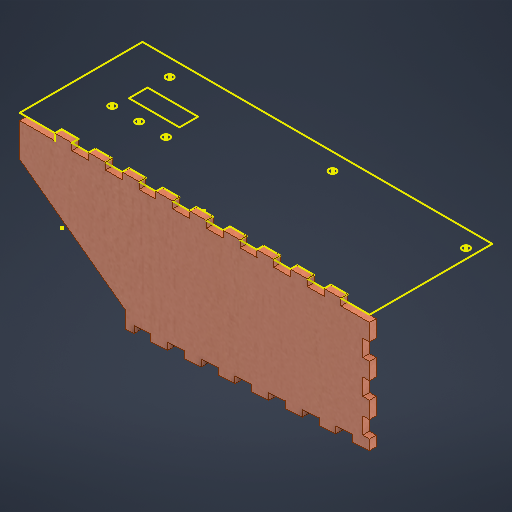
# Autodesk Inventor part: стульчак 2
Saved by Autodesk Inventor 2025 (Build 290162000, 162)
## iProperties
Created: 2025-01-28
Part Number: стульчак 2
Material: Древесина (орех)
Document SubType Name: Modeling
Designer: GameHD
Density: 0.55 g/cm^3
Appearance: Орех — натуральный — полированный
Author: GameHD
Autodesk Inventor part; units mm, degrees
ref_plane "YZ Plane" through (0, 0, 0) normal (1, 0, 0) x (0, 1, 0)
ref_plane "XZ Plane" through (0, 0, 0) normal (0, 1, 0) x (-1, 0, 0)
ref_plane "XY Plane" through (0, 0, 0) normal (0, 0, 1) x (1, 0, 0)
sketch "Эскиз1" plane through (0, 0, 0) normal (0, 0, 1) x (1, 0, 0)
  line L0 (105.5, -51) -> (-105.5, -51)
  line L1 (-105.5, -51) -> (-105.5, 51)
  line L2 (-105.5, 51) -> (105.5, 51)
  line L3 (105.5, 51) -> (105.5, -51)
  line L4 (105.5, -51) -> (-105.5, 51) construction
  line L5 (-105.5, -51) -> (105.5, 51) construction
  line L6 (105.5, 47) -> (-105.5, 47)
  line L7 (105.5, 47) -> (105.5, 51)
  line L8 (105.5, 51) -> (95.5, 51)
  line L9 (95.5, 51) -> (95.5, 47)
  line L10 (95.5, 47) -> (105.5, 47)
  line L11 (85.5, 51) -> (85.5, 47)
  line L12 (95.5, 51) -> (85.5, 51)
  line L13 (95.5, 47) -> (95.5, 51)
  line L14 (85.5, 47) -> (95.5, 47)
  line L15 (75.5, 51) -> (75.5, 47)
  line L16 (85.5, 51) -> (75.5, 51)
  line L17 (85.5, 47) -> (85.5, 51)
  line L18 (75.5, 47) -> (85.5, 47)
  line L19 (65.5, 51) -> (65.5, 47)
  line L20 (75.5, 51) -> (65.5, 51)
  line L21 (75.5, 47) -> (75.5, 51)
  line L22 (65.5, 47) -> (75.5, 47)
  line L23 (55.5, 51) -> (55.5, 47)
  line L24 (65.5, 51) -> (55.5, 51)
  line L25 (65.5, 47) -> (65.5, 51)
  line L26 (55.5, 47) -> (65.5, 47)
  line L27 (45.5, 51) -> (45.5, 47)
  line L28 (55.5, 51) -> (45.5, 51)
  line L29 (55.5, 47) -> (55.5, 51)
  line L30 (45.5, 47) -> (55.5, 47)
  line L31 (35.5, 51) -> (35.5, 47)
  line L32 (45.5, 51) -> (35.5, 51)
  line L33 (45.5, 47) -> (45.5, 51)
  line L34 (35.5, 47) -> (45.5, 47)
  line L35 (25.5, 51) -> (25.5, 47)
  line L36 (35.5, 51) -> (25.5, 51)
  line L37 (35.5, 47) -> (35.5, 51)
  line L38 (25.5, 47) -> (35.5, 47)
  line L39 (15.5, 51) -> (15.5, 47)
  line L40 (25.5, 51) -> (15.5, 51)
  line L41 (25.5, 47) -> (25.5, 51)
  line L42 (15.5, 47) -> (25.5, 47)
  line L43 (5.5, 51) -> (5.5, 47)
  line L44 (15.5, 51) -> (5.5, 51)
  line L45 (15.5, 47) -> (15.5, 51)
  line L46 (5.5, 47) -> (15.5, 47)
  line L47 (-4.5, 51) -> (-4.5, 47)
  line L48 (5.5, 51) -> (-4.5, 51)
  line L49 (5.5, 47) -> (5.5, 51)
  line L50 (-4.5, 47) -> (5.5, 47)
  line L51 (-14.5, 51) -> (-14.5, 47)
  line L52 (-4.5, 51) -> (-14.5, 51)
  line L53 (-4.5, 47) -> (-4.5, 51)
  line L54 (-14.5, 47) -> (-4.5, 47)
  line L55 (-24.5, 51) -> (-24.5, 47)
  line L56 (-14.5, 51) -> (-24.5, 51)
  line L57 (-14.5, 47) -> (-14.5, 51)
  line L58 (-24.5, 47) -> (-14.5, 47)
  line L59 (-34.5, 51) -> (-34.5, 47)
  line L60 (-24.5, 51) -> (-34.5, 51)
  line L61 (-24.5, 47) -> (-24.5, 51)
  line L62 (-34.5, 47) -> (-24.5, 47)
  line L63 (-44.5, 51) -> (-44.5, 47)
  line L64 (-34.5, 51) -> (-44.5, 51)
  line L65 (-34.5, 47) -> (-34.5, 51)
  line L66 (-44.5, 47) -> (-34.5, 47)
  line L67 (-54.5, 51) -> (-54.5, 47)
  line L68 (-44.5, 51) -> (-54.5, 51)
  line L69 (-44.5, 47) -> (-44.5, 51)
  line L70 (-54.5, 47) -> (-44.5, 47)
  line L71 (-64.5, 51) -> (-64.5, 47)
  line L72 (-54.5, 51) -> (-64.5, 51)
  line L73 (-54.5, 47) -> (-54.5, 51)
  line L74 (-64.5, 47) -> (-54.5, 47)
  line L75 (-74.5, 51) -> (-74.5, 47)
  line L76 (-64.5, 51) -> (-74.5, 51)
  line L77 (-64.5, 47) -> (-64.5, 51)
  line L78 (-74.5, 47) -> (-64.5, 47)
  line L79 (-84.5, 51) -> (-84.5, 47)
  line L80 (-74.5, 51) -> (-84.5, 51)
  line L81 (-74.5, 47) -> (-74.5, 51)
  line L82 (-84.5, 47) -> (-74.5, 47)
  line L83 (-84.5, 51) -> (-94.5, 51)
  line L84 (-84.5, 47) -> (-84.5, 51)
  line L85 (-94.5, 47) -> (-84.5, 47)
  line L86 (-94.5, 51) -> (-94.5, 49.2125)
  line L87 (-94.5, 49.2125) -> (-94.5, 47)
  point P0 (0, 0)
  point P1 (-105.5, 47)
  dimension "d0" = 211
  dimension "d1" = 102
  dimension "d2" = 4
  dimension "d3" = 10
  dimension "d4" = 4
  dimension "d5" = 10
  dimension "d6" = 4
  dimension "d7" = 10
  dimension "d8" = 4
  dimension "d9" = 10
  dimension "d10" = 4
  dimension "d11" = 10
  dimension "d12" = 4
  dimension "d13" = 10
  dimension "d14" = 4
  dimension "d15" = 10
  dimension "d16" = 4
  dimension "d17" = 10
  dimension "d18" = 4
  dimension "d19" = 10
  dimension "d20" = 4
  dimension "d21" = 10
  dimension "d22" = 4
  dimension "d23" = 10
  dimension "d24" = 4
  dimension "d25" = 10
  dimension "d26" = 4
  dimension "d27" = 10
  dimension "d28" = 4
  dimension "d29" = 10
  dimension "d30" = 4
  dimension "d31" = 10
  dimension "d32" = 4
  dimension "d33" = 10
  dimension "d34" = 4
  dimension "d35" = 10
  dimension "d36" = 4
  dimension "d37" = 10
  dimension "d38" = 4
  dimension "d39" = 10
  dimension "d40" = 10
  constraints: 174 end point, 40 parallel, 21 perpendicular, 2 horizontal, 2 midpoint, 1 collinear, 3 other
  measures "d0" distance of L1.end L3.start
  measures "d1" distance of L0.end L1.end
  measures "d2" distance of L10.start L8.end
  measures "d3" distance of L8.end L7.end
  measures "d4" distance of L14.start L11.start
  measures "d5" distance of L11.start L12.start
  measures "d6" distance of L15.end L15.start
  measures "d7" distance of L15.start L16.start
  measures "d8" distance of L19.end L19.start
  measures "d9" distance of L19.start L21.end
  measures "d10" distance of L23.end L23.start
  measures "d11" distance of L23.start L24.start
  measures "d12" distance of L27.end L27.start
  measures "d13" distance of L27.start L29.end
  measures "d14" distance of L34.start L32.end
  measures "d15" distance of L32.end L33.end
  measures "d16" distance of L38.start L35.start
  measures "d17" distance of L35.start L36.start
  measures "d18" distance of L39.end L39.start
  measures "d19" distance of L39.start L40.start
  measures "d20" distance of L46.start L44.end
  measures "d21" distance of L44.end L45.end
  measures "d22" distance of L50.start L48.end
  measures "d23" distance of L48.end L48.start
  measures "d24" distance of L54.start L51.start
  measures "d25" distance of L51.start L52.start
  measures "d26" distance of L55.end L55.start
  measures "d27" distance of L55.start L57.end
  measures "d28" distance of L62.start L60.end
  measures "d29" distance of L60.end L61.end
  measures "d30" distance of L66.start L63.start
  measures "d31" distance of L63.start L64.start
  measures "d32" distance of L67.end L67.start
  measures "d33" distance of L67.start L69.end
  measures "d34" distance of L74.start L71.start
  measures "d35" distance of L71.start L72.start
  measures "d36" distance of L78.start L75.start
  measures "d37" distance of L75.start L76.start
  measures "d38" distance of L82.start L79.start
  measures "d39" distance of L79.start L80.start
  measures "d40" distance of L83.end L84.end
extrude "Выдавливание1" add sketch "Эскиз1" along normal blind 4 contours L0 L1 L6 L3 | L6 L9 L2 L3 | L6 L15 L2 L11 | L79 L2 L75 L6 | L6 L23 L2 L19 | L71 L2 L67 L6 | L6 L31 L2 L27 | L63 L2 L59 L6 | L6 L39 L2 L35 | L55 L2 L51 L6 | L6 L47 L2 L43
sketch "Эскиз3" plane through (0, 0, 4) normal (0, 0, 1) x (1, 0, 0)
  line L0 (-105.5, -51) -> (105.5, -51) projected
  line L1 (-84.5, -51) -> (105.5, -51)
  line L2 (105.5, -51) -> (105.5, -83)
  line L3 (105.5, -83) -> (-84.5, -83)
  line L4 (-84.5, -83) -> (-84.5, -51)
  line L5 (105.5, -51) -> (-84.5, -51)
  line L6 (-84.5, -51) -> (-84.5, -19)
  line L7 (-84.5, -19) -> (105.5, -19)
  line L8 (105.5, -19) -> (105.5, -51)
  point P0 (0, 0)
  point P1 (105.5, -51)
  dimension "d45" = 190
  dimension "d46" = 32
  dimension "d47" = 190
  dimension "d48" = 32
  constraints: 16 end point, 4 parallel, 2 horizontal, 2 perpendicular
  measures "d45" distance of L2.end L3.end
  measures "d46" distance of L1.end L2.end
  measures "d47" distance of L6.end L7.end
  measures "d48" distance of L5.end L6.end
extrude "Выдавливание3" cut sketch "Эскиз3" against normal blind 10 contours L6 L7 L8 L0
sketch "Эскиз4" plane through (-84.5, 51, 0) normal (0, 1, 0) x (1, 0, 0)
  line L0 (10, 0) -> (10, -4) projected
  line L1 (187, -4) -> (187, 69) projected
  line L2 (187, 69) -> (-21, 69) projected
  line L3 (-21, -4) -> (-21, 69) projected
  circle A0 centre (102, 59) radius 2.1 projected
  circle A1 centre (5.1625, 59) radius 2.1 projected
  circle A2 centre (181.375, 59) radius 2.1 projected
  line L4 (10, 0) -> (0, 0) projected
  line L5 (0, 0) -> (0, -4) projected
  circle A3 centre (19, 27) radius 2.1 projected
  circle A4 centre (35, 27) radius 2.1 projected
  circle A5 centre (3, 27) radius 2.1 projected
  line L6 (4, 36) -> (4, 47) projected
  line L7 (4, 47) -> (34, 47) projected
  line L8 (34, 47) -> (34, 36) projected
  line L9 (34, 36) -> (4, 36) projected
  line L10 (-21, -4) -> (0, -4) projected
  line L11 (0, -4) -> (0, 0) projected
  line L12 (0, 0) -> (10, 0) projected
  line L13 (10, 0) -> (10, -4) projected
  line L14 (10, -4) -> (20, -4) projected
  line L15 (20, -4) -> (20, 0) projected
  line L16 (20, 0) -> (30, 0) projected
  line L17 (30, 0) -> (30, -4) projected
  line L18 (30, -4) -> (40, -4) projected
  line L19 (40, -4) -> (40, 0) projected
  line L20 (40, 0) -> (50, 0) projected
  line L21 (50, 0) -> (50, -4) projected
  line L22 (50, -4) -> (60, -4) projected
  line L23 (60, -4) -> (60, 0) projected
  line L24 (60, 0) -> (70, 0) projected
  line L25 (70, 0) -> (70, -4) projected
  line L26 (70, -4) -> (80, -4) projected
  line L27 (80, -4) -> (80, 0) projected
  line L28 (80, 0) -> (90, 0) projected
  line L29 (90, 0) -> (90, -4) projected
  line L30 (90, -4) -> (100, -4) projected
  line L31 (100, -4) -> (100, 0) projected
  line L32 (100, 0) -> (110, 0) projected
  line L33 (110, 0) -> (110, -4) projected
  line L34 (110, -4) -> (120, -4) projected
  line L35 (120, -4) -> (120, 0) projected
  line L36 (120, 0) -> (130, 0) projected
  line L37 (130, 0) -> (130, -4) projected
  line L38 (130, -4) -> (140, -4) projected
  line L39 (140, -4) -> (140, 0) projected
  line L40 (140, 0) -> (150, 0) projected
  line L41 (150, 0) -> (150, -4) projected
  line L42 (150, -4) -> (160, -4) projected
  line L43 (160, -4) -> (160, 0) projected
  line L44 (160, 0) -> (170, 0) projected
  line L45 (170, 0) -> (170, -4) projected
  line L46 (170, -4) -> (187, -4) projected
  point P0 (84.5, 0)
ref_plane "РабПлоскость1" through (-85.5, 47, -54) normal (0, -1, 0) x (1, 0, 0)
sketch "Эскиз5" plane through (-84.5, 47, 0) normal (-1, 0, 0) x (0, 0, -1)
  line L0 (0, -4) -> (0, 0) projected
  line L1 (-4, -4) -> (-4, 0) projected
  line L2 (0, -4) -> (-4, -4) projected
  line L3 (0, 0) -> (-4, 0) projected
  point P0 (0, 47)
ref_plane "РабПлоскость2" through (-85.5, 47, -54) normal (-1, 0, 0) x (0, 0, 1)
sketch "Эскиз6" plane through (0, 0, 4) normal (0, 0, 1) x (1, 0, 0)
  line L0 (-84.5, -19) -> (105.5, -19) projected
  line L1 (-84.5, -19) -> (-147.6375, -19)
  line L2 (-147.6375, -19) -> (-147.6375, -69.85)
  line L3 (-147.6375, -69.85) -> (-84.5, -69.85)
  line L4 (-84.5, -69.85) -> (-84.5, -19)
  point P0 (0, 0)
  constraints: 8 end point, 2 parallel, 1 horizontal, 1 perpendicular
extrude "Выдавливание6" cut sketch "Эскиз6" against normal blind 10
sketch "Эскиз7" plane through (95.5, 51, 0) normal (0, 1, 0) x (1, 0, 0)
  line L0 (10, 0) -> (0, 0) projected
  line L1 (0, 0) -> (0, -4) projected
  line L2 (10, -4) -> (0, -4) projected
  line L3 (10, 0) -> (10, -4) projected
  point P0 (-95.5, 0)
extrude "Выдавливание7" cut sketch "Эскиз7" against normal up to surface (4 mm away)
sketch "Эскиз8" plane through (85.5, 47, 0) normal (0, 1, 0) x (1, 0, 0)
  line L0 (17, -4) -> (17, 69) projected
  line L1 (20, 0) -> (20, -4) projected
  line L2 (20, -4) -> (0, -4) projected
  line L3 (0, 0) -> (20, 0) projected
  point P0 (-85.5, 0)
  point P1 (17, 0)
extrude "Выдавливание8" cut sketch "Эскиз8" against normal through all
sketch "Эскиз9" plane through (0, 0, 0) normal (0, 0, -1) x (-1, 0, 0)
  ellipse E0 centre (88.7842, -28.1226) end of major axis (84.7841, -28.1226) minor radius 4 (88.7842, -24.1226) -> (84.7841, -28.1226) ccw projected
  line L0 (84.7841, -28.1226) -> (84.7841, -65.1226) projected
  ellipse E1 centre (79.7838, -65.1226) end of major axis (84.7841, -65.1226) minor radius 5 (79.7838, -70.1226) -> (84.7841, -65.1226) ccw projected
  line L1 (79.7838, -70.1226) -> (66.4874, -70.1226) projected
  arc A0 (61.4874, -65.1226) -> (66.4874, -70.1226) centre (66.4874, -65.1226) ccw projected
  line L2 (61.4874, -65.1226) -> (61.4874, -28.1226) projected
  arc A1 (61.4874, -28.1226) -> (57.4874, -24.1226) centre (57.4874, -28.1226) ccw projected
  line L3 (48.6654, -24.1226) -> (57.4874, -24.1226) projected
  arc A2 (48.6654, -24.1226) -> (45.6654, -27.1226) centre (48.6654, -27.1226) ccw projected
  line L4 (45.6654, -70.1226) -> (45.6654, -27.1226) projected
  arc A3 (45.6654, -70.1226) -> (49.6654, -74.1226) centre (49.6654, -70.1226) ccw projected
  line L5 (49.6654, -74.1226) -> (125.5004, -74.1226) projected
  line L6 (125.5004, -70.1226) -> (125.5004, -74.1226) projected
  line L7 (109.5004, -70.1226) -> (125.5004, -70.1226) projected
  arc A4 (105.5004, -66.1226) -> (109.5004, -70.1226) centre (109.5004, -66.1226) ccw projected
  line L8 (105.5004, -24.1226) -> (105.5004, -66.1226) projected
  line L9 (88.7842, -24.1226) -> (105.5004, -24.1226) projected
  line L10 (105.5, 47) -> (105.5, -19) projected
  line L11 (105.5, 47) -> (105.5, 27)
  line L12 (105.5, 27) -> (42.8625, -19)
  line L13 (105.5, -19) -> (-102.5, -19) projected
  line L14 (-102.5, -19) -> (105.5, -19) projected
  line L15 (105.5004, 27) -> (105.5004, -13) projected
  line L16 (105.5, 47) -> (105.5, -19) projected
  point P0 (0, 0)
  dimension "d61" = 20
  constraints: 4 end point, 2 point on line, 2 other
  measures "d61" distance of L10.start L11.end
extrude "Выдавливание9" cut sketch "Эскиз9" against normal blind 10 contours L10 L13 L12
sketch "Эскиз10" plane through (0, 0, 4) normal (0, 0, 1) x (1, 0, 0)
  line L0 (102.5, 47) -> (102.5, -19) projected
  line L1 (102.5, -19) -> (92.5, -19)
  line L2 (92.5, -19) -> (92.5, -15)
  line L3 (92.5, -15) -> (102.5, -15)
  line L4 (102.5, -15) -> (102.5, -19)
  line L5 (92.5, -19) -> (82.5, -19)
  line L6 (82.5, -19) -> (82.5, -15)
  line L7 (82.5, -15) -> (92.5, -15)
  line L8 (92.5, -15) -> (92.5, -19)
  line L9 (82.5, -19) -> (72.5, -19)
  line L10 (72.5, -19) -> (72.5, -15)
  line L11 (72.5, -15) -> (82.5, -15)
  line L12 (82.5, -15) -> (82.5, -19)
  line L13 (72.5, -19) -> (62.5, -19)
  line L14 (62.5, -19) -> (62.5, -15)
  line L15 (62.5, -15) -> (72.5, -15)
  line L16 (72.5, -15) -> (72.5, -19)
  line L17 (62.5, -19) -> (52.5, -19)
  line L18 (52.5, -19) -> (52.5, -15)
  line L19 (52.5, -15) -> (62.5, -15)
  line L20 (62.5, -15) -> (62.5, -19)
  line L21 (52.5, -19) -> (42.5, -19)
  line L22 (42.5, -19) -> (42.5, -15)
  line L23 (42.5, -15) -> (52.5, -15)
  line L24 (52.5, -15) -> (52.5, -19)
  line L25 (42.5, -19) -> (32.5, -19)
  line L26 (32.5, -19) -> (32.5, -15)
  line L27 (32.5, -15) -> (42.5, -15)
  line L28 (42.5, -15) -> (42.5, -19)
  line L29 (32.5, -19) -> (22.5, -19)
  line L30 (22.5, -19) -> (22.5, -15)
  line L31 (22.5, -15) -> (32.5, -15)
  line L32 (32.5, -15) -> (32.5, -19)
  line L33 (22.5, -19) -> (12.5, -19)
  line L34 (12.5, -19) -> (12.5, -15)
  line L35 (12.5, -15) -> (22.5, -15)
  line L36 (22.5, -15) -> (22.5, -19)
  line L37 (12.5, -19) -> (2.5, -19)
  line L38 (2.5, -19) -> (2.5, -15)
  line L39 (2.5, -15) -> (12.5, -15)
  line L40 (12.5, -15) -> (12.5, -19)
  line L41 (2.5, -19) -> (-7.5, -19)
  line L42 (-7.5, -19) -> (-7.5, -15)
  line L43 (-7.5, -15) -> (2.5, -15)
  line L44 (2.5, -15) -> (2.5, -19)
  line L45 (-7.5, -19) -> (-17.5, -19)
  line L46 (-17.5, -19) -> (-17.5, -15)
  line L47 (-17.5, -15) -> (-7.5, -15)
  line L48 (-7.5, -15) -> (-7.5, -19)
  line L49 (-17.5, -19) -> (-27.5, -19)
  line L50 (-27.5, -19) -> (-27.5, -15)
  line L51 (-27.5, -15) -> (-17.5, -15)
  line L52 (-17.5, -15) -> (-17.5, -19)
  line L53 (-27.5, -19) -> (-37.5, -19)
  line L54 (-37.5, -19) -> (-37.5, -15)
  line L55 (-37.5, -15) -> (-27.5, -15)
  line L56 (-27.5, -15) -> (-27.5, -19)
  point P0 (0, 0)
  dimension "d64" = 10
  dimension "d65" = 4
  dimension "d66" = 10
  dimension "d67" = 4
  dimension "d68" = 10
  dimension "d69" = 4
  dimension "d70" = 10
  dimension "d71" = 4
  dimension "d72" = 10
  dimension "d73" = 4
  dimension "d74" = 10
  dimension "d75" = 4
  dimension "d76" = 10
  dimension "d77" = 4
  dimension "d78" = 10
  dimension "d79" = 4
  dimension "d80" = 10
  dimension "d81" = 4
  dimension "d82" = 10
  dimension "d83" = 4
  dimension "d84" = 10
  dimension "d85" = 4
  dimension "d86" = 10
  dimension "d87" = 4
  dimension "d88" = 10
  dimension "d89" = 4
  dimension "d90" = 10
  dimension "d91" = 4
  constraints: 112 end point, 28 parallel, 14 horizontal, 14 perpendicular
  measures "d64" distance of L2.end L3.end
  measures "d65" distance of L1.end L2.end
  measures "d66" distance of L7.start L7.end
  measures "d67" distance of L6.start L7.start
  measures "d68" distance of L11.start L11.end
  measures "d69" distance of L10.start L11.start
  measures "d70" distance of L15.start L15.end
  measures "d71" distance of L14.start L15.start
  measures "d72" distance of L19.start L19.end
  measures "d73" distance of L18.start L19.start
  measures "d74" distance of L23.start L23.end
  measures "d75" distance of L22.start L23.start
  measures "d76" distance of L27.start L27.end
  measures "d77" distance of L26.start L27.start
  measures "d78" distance of L31.start L31.end
  measures "d79" distance of L30.start L31.start
  measures "d80" distance of L35.start L35.end
  measures "d81" distance of L34.start L35.start
  measures "d82" distance of L39.start L39.end
  measures "d83" distance of L38.start L39.start
  measures "d84" distance of L43.start L43.end
  measures "d85" distance of L42.start L43.start
  measures "d86" distance of L47.start L47.end
  measures "d87" distance of L46.start L47.start
  measures "d88" distance of L51.start L51.end
  measures "d89" distance of L50.start L51.start
  measures "d90" distance of L55.start L55.end
  measures "d91" distance of L54.start L55.start
extrude "Выдавливание10" cut sketch "Эскиз10" against normal blind 10 contours L2 L5 L6 L7 | L10 L13 L14 L15 | L18 L21 L22 L23 | L26 L29 L30 L31 | L34 L37 L38 L39 | L42 L45 L46 L47 | L50 L53 L54 L55
sketch "Эскиз12" plane through (0, 0, 4) normal (0, 0, 1) x (1, 0, 0)
  line L0 (2.5, -19) -> (2.5, -15) projected
  line L1 (2.5, -15) -> (12.5, -15) projected
  line L2 (12.5, -15) -> (12.5, -19) projected
  line L3 (12.5, -19) -> (22.5, -19) projected
  line L4 (22.5, -19) -> (22.5, -15) projected
  line L5 (22.5, -15) -> (32.5, -15) projected
  line L6 (32.5, -15) -> (32.5, -19) projected
  line L7 (32.5, -19) -> (42.5, -19) projected
  line L8 (42.5, -19) -> (42.5, -15) projected
  line L9 (42.5, -15) -> (52.5, -15) projected
  line L10 (52.5, -15) -> (52.5, -19) projected
  line L11 (52.5, -19) -> (62.5, -19) projected
  line L12 (62.5, -19) -> (62.5, -15) projected
  line L13 (62.5, -15) -> (72.5, -15) projected
  line L14 (72.5, -15) -> (72.5, -19) projected
  line L15 (72.5, -19) -> (82.5, -19) projected
  line L16 (82.5, -19) -> (82.5, -15) projected
  line L17 (82.5, -15) -> (92.5, -15) projected
  line L18 (92.5, -15) -> (92.5, -19) projected
  line L19 (92.5, -19) -> (102.5, -19) projected
  line L20 (102.5, -19) -> (102.5, 47) projected
  line L21 (102.5, 47) -> (85.5, 47) projected
  line L22 (85.5, 47) -> (85.5, 51) projected
  line L23 (85.5, 51) -> (75.5, 51) projected
  line L24 (75.5, 51) -> (75.5, 47) projected
  line L25 (75.5, 47) -> (65.5, 47) projected
  line L26 (65.5, 47) -> (65.5, 51) projected
  line L27 (65.5, 51) -> (55.5, 51) projected
  line L28 (55.5, 51) -> (55.5, 47) projected
  line L29 (55.5, 47) -> (45.5, 47) projected
  line L30 (45.5, 47) -> (45.5, 51) projected
  line L31 (45.5, 51) -> (35.5, 51) projected
  line L32 (35.5, 51) -> (35.5, 47) projected
  line L33 (35.5, 47) -> (25.5, 47) projected
  line L34 (25.5, 47) -> (25.5, 51) projected
  line L35 (25.5, 51) -> (15.5, 51) projected
  line L36 (15.5, 51) -> (15.5, 47) projected
  line L37 (15.5, 47) -> (5.5, 47) projected
  line L38 (5.5, 47) -> (5.5, 51) projected
  line L39 (5.5, 51) -> (-4.5, 51) projected
  line L40 (-4.5, 51) -> (-4.5, 47) projected
  line L41 (-4.5, 47) -> (-14.5, 47) projected
  line L42 (-14.5, 47) -> (-14.5, 51) projected
  line L43 (-14.5, 51) -> (-24.5, 51) projected
  line L44 (-24.5, 51) -> (-24.5, 47) projected
  line L45 (-24.5, 47) -> (-34.5, 47) projected
  line L46 (-34.5, 47) -> (-34.5, 51) projected
  line L47 (-34.5, 51) -> (-44.5, 51) projected
  line L48 (-44.5, 51) -> (-44.5, 47) projected
  line L49 (-44.5, 47) -> (-54.5, 47) projected
  line L50 (-54.5, 47) -> (-54.5, 51) projected
  line L51 (-54.5, 51) -> (-64.5, 51) projected
  line L52 (-64.5, 51) -> (-64.5, 47) projected
  line L53 (-64.5, 47) -> (-74.5, 47) projected
  line L54 (-74.5, 47) -> (-74.5, 51) projected
  line L55 (-74.5, 51) -> (-84.5, 51) projected
  line L56 (-84.5, 51) -> (-84.5, 47) projected
  line L57 (-84.5, 47) -> (-105.5, 47) projected
  line L58 (-105.5, 47) -> (-105.5, 27) projected
  line L59 (-105.5, 27) -> (-42.8625, -19) projected
  line L60 (-42.8625, -19) -> (-37.5, -19) projected
  line L61 (-37.5, -19) -> (-37.5, -15) projected
  line L62 (-37.5, -15) -> (-27.5, -15) projected
  line L63 (-27.5, -15) -> (-27.5, -19) projected
  line L64 (-27.5, -19) -> (-17.5, -19) projected
  line L65 (-17.5, -19) -> (-17.5, -15) projected
  line L66 (-17.5, -15) -> (-7.5, -15) projected
  line L67 (-7.5, -15) -> (-7.5, -19) projected
  line L68 (-7.5, -19) -> (2.5, -19) projected
  line L69 (102.5, -15) -> (102.5, -29)
  line L70 (102.5, -29) -> (-42.8625, -29)
  line L71 (-42.8625, -29) -> (-42.8625, -25)
  line L72 (-42.8625, -25) -> (102.5, -15)
  line L73 (102.5, -15) -> (102.5, -19)
  line L74 (-42.8625, -19) -> (-42.8625, -25)
  line L75 (-37.5, -19) -> (-37.5, -28.6311)
  line L76 (-17.5, -19) -> (-27.5, -19) projected
  line L77 (-27.5, -19) -> (-27.5, -27.9432)
  line L78 (-17.5, -19) -> (-17.5, -27.2552)
  line L79 (-7.5, -19) -> (-7.5, -26.5673)
  line L80 (-7.5, -19) -> (2.5, -19) projected
  line L81 (2.5, -19) -> (2.5, -25.8794)
  line L82 (22.5, -19) -> (12.5, -19) projected
  line L83 (12.5, -19) -> (12.5, -25.1914)
  line L84 (22.5, -19) -> (22.5, -24.5035)
  line L85 (32.5, -19) -> (32.5, -23.8155)
  line L86 (52.5, -19) -> (52.5, -22.4397)
  line L87 (62.5, -19) -> (52.5, -19) projected
  line L88 (62.5, -19) -> (62.5, -21.7517)
  line L89 (72.5, -19) -> (72.5, -21.0638)
  line L90 (82.5, -19) -> (82.5, -20.3759)
  line L91 (92.5, -19) -> (92.5, -19.6879)
  line L92 (42.5, -19) -> (42.5, -23.1276)
  line L93 (102.5, -15) -> (102.5, -19)
  line L94 (102.5, 47) -> (102.5, -19) projected
  line L95 (102.5, -19) -> (-42.8625, -29)
  point P0 (0, 0)
  point P1 (82.5, -16.3759)
  point P2 (92.5, -15.6879)
  point P3 (62.5, -17.7517)
  point P4 (72.5, -17.0638)
  point P5 (42.5, -19.1276)
  point P6 (52.5, -18.4397)
  point P7 (22.5, -20.5035)
  point P8 (32.5, -19.8155)
  point P9 (2.5, -21.8794)
  point P10 (12.5, -21.1914)
  point P11 (-37.5, -24.6311)
  point P12 (-27.5, -23.9432)
  point P13 (-17.5, -23.2552)
  point P14 (-7.5, -22.5673)
  dimension "d94" = 14
  dimension "d95" = 4
  dimension "d98" = 4
  constraints: 44 end point, 12 vertical, 6 perpendicular, 2 collinear, 1 point on line
  measures "d94" distance of L69.start L69.end
  measures "d95" distance of L70.end L71.end
  measures "d98" distance of L69.start L19.end
extrude "Выдавливание11" add sketch "Эскиз12" against normal up to surface (4 mm away) contours L68 L67 L66 L65 L64 L63 L62 L61 L60 L59 L58 L57 L56 L55 L54 L53 L52 L51 L50 L49 L48 L47 L46 L45 L44 L43 L42 L41 L40 L39 L38 L37 L36 L35 L34 L33 L32 L31 L30 L29 L28 L27 L26 L25 L24 L23 L22 L21 L20 L72 L18 L17 L16 L14 L13 L12 L10 L9 L8 L7 L6 L5 L4 L3 L2 L1 L0 | L81 L72 L79 L68 | L0 L1 L2 L83 L72 L81 | L79 L72 L78 L65 L66 L67 | L81 L95 L79 L72 | L83 L3 L84 L72 | L72 L84 L95 L83 | L78 L95 L77 L72 | L72 L77 L64 L78 | L84 L4 L5 L6 L85 L72 | L72 L75 L61 L62 L63 L77 | L85 L7 L92 L72 | L72 L92 L95 L85 | L75 L95 L71 L72 | L72 L74 L60 L75 | L92 L8 L9 L10 L72 | L11 L88 L95 L86 | L12 L13 L14 L72 | L95 L91 L19 | L15 L90 L95 L89 | L16 L17 L18 L72
sketch "Эскиз13" plane through (0, 0, 4) normal (0, 0, 1) x (1, 0, 0)
  line L0 (85.5, 47) -> (102.5, 47) projected
  line L1 (102.5, 47) -> (98.5, 47)
  line L2 (98.5, 47) -> (98.5, 37)
  line L3 (98.5, 37) -> (102.5, 37)
  line L4 (102.5, 37) -> (102.5, 47)
  line L5 (102.5, 37) -> (98.5, 37)
  line L6 (98.5, 37) -> (98.5, 27)
  line L7 (98.5, 27) -> (102.5, 27)
  line L8 (102.5, 27) -> (102.5, 37)
  line L9 (102.5, 27) -> (98.5, 27)
  line L10 (98.5, 27) -> (98.5, 17)
  line L11 (98.5, 17) -> (102.5, 17)
  line L12 (102.5, 17) -> (102.5, 27)
  line L13 (102.5, 17) -> (98.5, 17)
  line L14 (98.5, 17) -> (98.5, 7)
  line L15 (98.5, 7) -> (102.5, 7)
  line L16 (102.5, 7) -> (102.5, 17)
  line L17 (102.5, 7) -> (98.5, 7)
  line L18 (98.5, 7) -> (98.5, -3)
  line L19 (98.5, -3) -> (102.5, -3)
  line L20 (102.5, -3) -> (102.5, 7)
  line L21 (102.5, -3) -> (98.5, -3)
  line L22 (98.5, -3) -> (98.5, -13)
  line L23 (98.5, -13) -> (102.5, -13)
  line L24 (102.5, -13) -> (102.5, -3)
  point P0 (0, 0)
  dimension "d99" = 4
  dimension "d100" = 10
  dimension "d101" = 4
  dimension "d102" = 10
  dimension "d103" = 4
  dimension "d104" = 10
  dimension "d105" = 4
  dimension "d106" = 10
  dimension "d107" = 4
  dimension "d108" = 10
  dimension "d109" = 4
  dimension "d110" = 10
  constraints: 48 end point, 12 parallel, 6 horizontal, 6 perpendicular
  measures "d99" distance of L3.end L2.end
  measures "d100" distance of L2.end L1.end
  measures "d101" distance of L7.end L6.end
  measures "d102" distance of L6.end L5.end
  measures "d103" distance of L11.end L10.end
  measures "d104" distance of L10.end L9.end
  measures "d105" distance of L15.end L14.end
  measures "d106" distance of L14.end L13.end
  measures "d107" distance of L19.end L18.end
  measures "d108" distance of L18.end L17.end
  measures "d109" distance of L23.end L22.end
  measures "d110" distance of L22.end L21.end
extrude "Выдавливание12" cut sketch "Эскиз13" against normal blind 10 contours L3 L8 L7 L6 | L11 L16 L15 L14 | L19 L24 L23 L22
